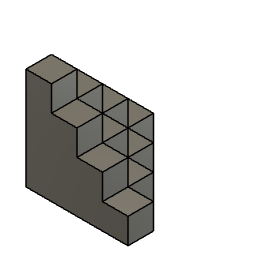
EXTRUDES&PLANES (Autodesk Fusion 360 design; units mm, degrees)
Autodesk Fusion 360 part; units mm, degrees
sketch "Sketch1" plane through (0, 0, 0) normal (0, 1, 0) x (1, 0, 0)
  line L0 (0, 0) -> (20, 0)
  line L1 (0, 20) -> (0, 0)
  line L2 (20, 0) -> (40, 0)
  line L3 (40, 0) -> (60, 0)
  line L4 (60, 0) -> (80, 0)
  line L5 (80, 20) -> (60, 20)
  line L6 (80, 0) -> (80, 20)
  line L7 (0, 40) -> (0, 20)
  line L8 (0, 60) -> (0, 40)
  line L9 (20, 80) -> (0, 80)
  line L10 (20, 80) -> (20, 60)
  line L11 (0, 80) -> (0, 60)
  line L12 (40, 60) -> (20, 60)
  line L13 (40, 40) -> (40, 60)
  line L14 (60, 40) -> (40, 40)
  line L15 (60, 40) -> (60, 20)
  point P0 (20, 0)
  point P1 (40, 0)
  point P2 (60, 0)
  dimension "d1" = 20
  dimension "d2" = 20
  constraint horizontal L0
  constraint vertical L1
  constraint coincident L0.start L1.end
  measures "d1" distance of L0.start P0
  measures "d2" distance of L0.start L1.start
extrude "Extrude1" add sketch "Sketch1" along normal blind 20
sketch "Sketch2" plane through (0, 20, 0) normal (0, 1, 0) x (-1, 0, 0)
  line L0 (-40, -40) -> (-40, -60)
  line L1 (-40, -60) -> (-20, -60)
  line L2 (-20, -60) -> (-20, -80)
  line L3 (-20, -80) -> (0, -80)
  line L4 (0, -80) -> (0, 0)
  line L5 (0, 0) -> (-80, 0)
  line L6 (-80, 0) -> (-80, -20)
  line L7 (-80, -20) -> (-60, -20)
  line L8 (-60, -20) -> (-60, -40)
  line L9 (-60, -40) -> (-40, -40)
  line L10 (0, 0) -> (-20, 0)
  line L11 (-20, -40) -> (-20, -60)
  line L12 (-20, -60) -> (0, -60)
  line L13 (0, -60) -> (0, 0)
  line L14 (-20, 0) -> (-40, 0)
  line L15 (-40, -40) -> (-20, -40)
  line L16 (-40, 0) -> (-60, 0)
  line L17 (-60, 0) -> (-60, -20)
  line L18 (-60, -20) -> (-40, -20)
  line L19 (-40, -20) -> (-40, -40)
  dimension "d21" = 20
  dimension "d22" = 60
  dimension "d23" = 20
  dimension "d24" = 40
  dimension "d25" = 20
  dimension "d26" = 20
  constraint horizontal L10
  constraint vertical L11
  constraint horizontal L12
  constraint vertical L13
  constraint coincident L4.end L5.start
  constraint horizontal L14
  constraint horizontal L15
  constraint horizontal L16
  constraint vertical L17
  constraint horizontal L18
  measures "d21" distance of L4.end L10.end
  measures "d22" distance of L4.end L12.end
  measures "d23" distance of L10.end L14.end
  measures "d24" distance of L10.end L11.start
  measures "d25" distance of L14.end L16.end
  measures "d26" distance of L14.end L18.end
extrude "Extrude2" add sketch "Sketch2" along normal blind 20 contours L4 L5 L10 L11 L12 L13 L14 L15 L16 L17 L18 L19
sketch "Sketch3" plane through (0, 40, 0) normal (0, 1, 0) x (-1, 0, 0)
  line L0 (-40, -20) -> (-40, -40)
  line L1 (-40, -40) -> (-20, -40)
  line L2 (-20, -40) -> (-20, -60)
  line L3 (-20, -60) -> (0, -60)
  line L4 (0, -60) -> (0, 0)
  line L5 (0, 0) -> (-60, 0)
  line L6 (-60, 0) -> (-60, -20)
  line L7 (-60, -20) -> (-40, -20)
  line L8 (0, 0) -> (-40, 0)
  line L9 (-40, 0) -> (-40, -20)
  line L10 (-40, -20) -> (-20, -20)
  line L11 (0, -20) -> (0, 0)
  line L12 (-20, -20) -> (-20, -40)
  line L13 (-20, -40) -> (0, -40)
  line L14 (0, -40) -> (0, -20)
  dimension "d29" = 40
  dimension "d30" = 20
  dimension "d31" = 20
  dimension "d32" = 20
  constraint horizontal L8
  constraint vertical L9
  constraint horizontal L10
  constraint vertical L11
  constraint coincident L4.end L5.start
  constraint vertical L12
  constraint horizontal L13
  constraint vertical L14
  measures "d29" distance of L4.end L8.end
  measures "d30" distance of L4.end L11.start
  measures "d31" distance of L11.start L10.end
  measures "d32" distance of L11.start L13.end
extrude "Extrude3" add sketch "Sketch3" along normal blind 20 contours L4 L5 L8 L9 L10 L11 L12 L13 L14
sketch "Sketch4" plane through (0, 60, 0) normal (0, 1, 0) x (-1, 0, 0)
  line L0 (0, -40) -> (0, 0)
  line L1 (0, 0) -> (-40, 0)
  line L2 (-40, 0) -> (-40, -20)
  line L3 (-40, -20) -> (-20, -20)
  line L4 (-20, -20) -> (-20, -40)
  line L5 (-20, -40) -> (0, -40)
  line L6 (0, 0) -> (-20, 0)
  line L7 (-20, 0) -> (-20, -20)
  line L8 (-20, -20) -> (0, -20)
  line L9 (0, -20) -> (0, 0)
  dimension "d35" = 20
  dimension "d36" = 20
  constraint horizontal L6
  constraint vertical L7
  constraint horizontal L8
  constraint vertical L9
  constraint coincident L0.end L1.start
  measures "d35" distance of L0.end L6.end
  measures "d36" distance of L0.end L8.end
extrude "Extrude4" add sketch "Sketch4" along normal blind 20 contours L0 L1 L6 L7 L8 L9
shell "Shell1" thickness 4 removed faces 1 at (20, 0, -33.3333)
